Autodesk Fusion 360 part; units mm, degrees
(part 7 of 12)
  line L124 (13.462, -40.1221) -> (13.462, -36.3221)
  line L125 (17.262, -40.1221) -> (13.462, -40.1221)
  line L126 (13.462, -36.3221) -> (17.262, -36.3221)
  line L127 (17.262, -36.3221) -> (17.262, -40.1221)
  line L128 (52.9466, -41.1381) -> (49.1466, -41.1381)
  line L129 (49.1466, -41.1381) -> (49.1466, -37.3381)
  line L130 (49.1466, -37.3381) -> (52.9466, -37.3381)
  line L131 (52.9466, -37.3381) -> (52.9466, -41.1381)
  line L132 (-185.9511, -63.3791) -> (-185.9511, -67.1791)
  line L133 (-185.9511, -67.1791) -> (-189.7511, -67.1791)
  line L134 (-189.7511, -63.3791) -> (-185.9511, -63.3791)
  line L135 (-189.7511, -67.1791) -> (-189.7511, -63.3791)
  line L136 (-155.9511, -67.1791) -> (-159.7511, -67.1791)
  line L137 (-159.7511, -67.1791) -> (-159.7511, -63.3791)
  line L138 (-155.9511, -63.3791) -> (-155.9511, -67.1791)
  line L139 (-159.7511, -63.3791) -> (-155.9511, -63.3791)
  line L140 (-125.9511, -67.1791) -> (-129.7511, -67.1791)
  line L141 (-125.9511, -63.3791) -> (-125.9511, -67.1791)
  line L142 (-129.7511, -67.1791) -> (-129.7511, -63.3791)
  line L143 (-129.7511, -63.3791) -> (-125.9511, -63.3791)
  line L144 (-99.7511, -67.1791) -> (-99.7511, -63.3791)
  line L145 (-95.9511, -67.1791) -> (-99.7511, -67.1791)
  line L146 (-99.7511, -63.3791) -> (-95.9511, -63.3791)
  line L147 (-95.9511, -63.3791) -> (-95.9511, -67.1791)
  line L148 (-69.7511, -63.3791) -> (-65.9511, -63.3791)
  line L149 (-65.9511, -63.3791) -> (-65.9511, -67.1791)
  line L150 (-69.7511, -67.1791) -> (-69.7511, -63.3791)
  line L151 (-65.9511, -67.1791) -> (-69.7511, -67.1791)
  line L152 (-35.9511, -63.3791) -> (-35.9511, -67.1791)
  line L153 (-39.7511, -63.3791) -> (-35.9511, -63.3791)
  line L154 (-39.7511, -67.1791) -> (-39.7511, -63.3791)
  line L155 (-35.9511, -67.1791) -> (-39.7511, -67.1791)
  line L156 (6.975, -64.3891) -> (6.975, -68.1891)
  line L157 (3.175, -68.1891) -> (3.175, -64.3891)
  line L158 (3.175, -64.3891) -> (6.975, -64.3891)
  line L159 (6.975, -68.1891) -> (3.175, -68.1891)
  line L160 (-174.6989, -98.2882) -> (-178.4989, -98.2882)
  line L161 (-178.4989, -98.2882) -> (-178.4989, -94.4882)
  line L162 (-178.4989, -94.4882) -> (-174.6989, -94.4882)
  line L163 (-174.6989, -94.4882) -> (-174.6989, -98.2882)
  line L164 (52.0701, -75.5551) -> (52.0701, -71.7551)
  line L165 (55.8701, -71.7551) -> (55.8701, -75.5551)
  line L166 (55.8701, -75.5551) -> (52.0701, -75.5551)
  line L167 (52.0701, -71.7551) -> (55.8701, -71.7551)
  line L168 (-144.2823, -98.2882) -> (-148.0823, -98.2882)
  line L169 (-144.2823, -94.4882) -> (-144.2823, -98.2882)
  line L170 (-148.0823, -94.4882) -> (-144.2823, -94.4882)
  line L171 (-148.0823, -98.2882) -> (-148.0823, -94.4882)
  line L172 (-113.8658, -94.4882) -> (-113.8658, -98.2882)
  line L173 (-117.6658, -94.4882) -> (-113.8658, -94.4882)
  line L174 (-113.8658, -98.2882) -> (-117.6658, -98.2882)
  line L175 (-117.6658, -98.2882) -> (-117.6658, -94.4882)
  line L176 (-83.4492, -98.2882) -> (-87.2492, -98.2882)
  line L177 (-83.4492, -94.4882) -> (-83.4492, -98.2882)
  line L178 (-87.2492, -94.4882) -> (-83.4492, -94.4882)
  line L179 (-87.2492, -98.2882) -> (-87.2492, -94.4882)
  line L180 (-53.0326, -94.4882) -> (-53.0326, -98.2882)
  line L181 (-56.8326, -94.4882) -> (-53.0326, -94.4882)
  line L182 (-56.8326, -98.2882) -> (-56.8326, -94.4882)
  line L183 (-53.0326, -98.2882) -> (-56.8326, -98.2882)
  line L184 (-22.6161, -94.4882) -> (-22.6161, -98.2882)
  line L185 (-26.4161, -94.4882) -> (-22.6161, -94.4882)
  line L186 (-22.6161, -98.2882) -> (-26.4161, -98.2882)
  line L187 (-26.4161, -98.2882) -> (-26.4161, -94.4882)
  line L188 (7.737, -98.3894) -> (3.937, -98.3894)
  line L189 (3.937, -98.3894) -> (3.937, -94.5894)
  line L190 (7.737, -94.5894) -> (7.737, -98.3894)
  line L191 (3.937, -94.5894) -> (7.737, -94.5894)
  line L192 (-155.2293, -124.9242) -> (-155.2293, -128.7242)
  line L193 (-155.2293, -128.7242) -> (-159.0293, -128.7242)
  line L194 (-159.0293, -124.9242) -> (-155.2293, -124.9242)
  line L195 (-159.0293, -128.7242) -> (-159.0293, -124.9242)
  line L196 (-116.37, -124.9242) -> (-112.57, -124.9242)
  line L197 (-112.57, -124.9242) -> (-112.57, -128.7242)
  line L198 (-112.57, -128.7242) -> (-116.37, -128.7242)
  line L199 (-116.37, -128.7242) -> (-116.37, -124.9242)
  line L200 (-82.57, -128.7242) -> (-86.37, -128.7242)
  line L201 (-86.37, -128.7242) -> (-86.37, -124.9242)
  line L202 (-86.37, -124.9242) -> (-82.57, -124.9242)
  line L203 (-82.57, -124.9242) -> (-82.57, -128.7242)
  line L204 (-52.57, -128.7242) -> (-56.37, -128.7242)
  line L205 (-56.37, -128.7242) -> (-56.37, -124.9242)
  line L206 (-52.57, -124.9242) -> (-52.57, -128.7242)
  line L207 (-56.37, -124.9242) -> (-52.57, -124.9242)
  line L208 (-22.57, -124.9242) -> (-22.57, -128.7242)
  line L209 (-22.57, -128.7242) -> (-26.37, -128.7242)
  line L210 (-26.37, -124.9242) -> (-22.57, -124.9242)
  line L211 (-26.37, -128.7242) -> (-26.37, -124.9242)
  line L212 (3.63, -124.9242) -> (7.43, -124.9242)
  line L213 (7.43, -128.7242) -> (3.63, -128.7242)
  line L214 (7.43, -124.9242) -> (7.43, -128.7242)
  line L215 (3.63, -128.7242) -> (3.63, -124.9242)
  line L216 (33.63, -124.9242) -> (37.43, -124.9242)
  line L217 (37.43, -128.7242) -> (33.63, -128.7242)
  line L218 (33.63, -128.7242) -> (33.63, -124.9242)
  line L219 (37.43, -124.9242) -> (37.43, -128.7242)
  line L220 (66.8401, 26.2001) -> (66.8401, 24.6001)
  line L221 (65.2401, 24.6001) -> (65.2401, 26.2001)
  line L222 (65.2401, 26.2001) -> (66.8401, 26.2001)
  line L223 (66.8401, 24.6001) -> (65.2401, 24.6001)
  line L224 (66.8401, 24.6001) -> (65.2401, 24.6001)
  line L225 (65.2401, 24.6001) -> (65.2401, 26.2001)
  line L226 (65.2401, 26.2001) -> (66.8401, 26.2001)
  line L227 (66.8401, 26.2001) -> (66.8401, 24.6001)
  line L228 (65.2401, 24.6001) -> (65.2401, 26.2001)
  line L229 (66.8401, 26.2001) -> (66.8401, 24.6001)
  line L230 (65.2401, 26.2001) -> (66.8401, 26.2001)
  line L231 (66.8401, 24.6001) -> (65.2401, 24.6001)
  arc A292 (65.2401, 22.86) -> (66.8401, 22.86) centre (66.0401, 22.86) ccw
  arc A293 (66.8401, 22.86) -> (65.2401, 22.86) centre (66.0401, 22.86) ccw
  arc A294 (65.2401, 22.86) -> (66.8401, 22.86) centre (66.0401, 22.86) ccw
  arc A295 (66.8401, 22.86) -> (65.2401, 22.86) centre (66.0401, 22.86) ccw
  arc A296 (66.8401, 22.86) -> (65.2401, 22.86) centre (66.0401, 22.86) ccw
  arc A297 (65.2401, 22.86) -> (66.8401, 22.86) centre (66.0401, 22.86) ccw
  arc A298 (66.8401, 20.32) -> (65.2401, 20.32) centre (66.0401, 20.32) ccw
  arc A299 (65.2401, 20.32) -> (66.8401, 20.32) centre (66.0401, 20.32) ccw
  arc A300 (65.2401, 20.32) -> (66.8401, 20.32) centre (66.0401, 20.32) ccw
  arc A301 (66.8401, 20.32) -> (65.2401, 20.32) centre (66.0401, 20.32) ccw
  arc A302 (65.2401, 20.32) -> (66.8401, 20.32) centre (66.0401, 20.32) ccw
  arc A303 (66.8401, 20.32) -> (65.2401, 20.32) centre (66.0401, 20.32) ccw
  arc A304 (65.2401, 17.78) -> (66.8401, 17.78) centre (66.0401, 17.78) ccw
  arc A305 (66.8401, 17.78) -> (65.2401, 17.78) centre (66.0401, 17.78) ccw
  arc A306 (65.2401, 17.78) -> (66.8401, 17.78) centre (66.0401, 17.78) ccw
  arc A307 (66.8401, 17.78) -> (65.2401, 17.78) centre (66.0401, 17.78) ccw
  arc A308 (66.8401, 17.78) -> (65.2401, 17.78) centre (66.0401, 17.78) ccw
  arc A309 (65.2401, 17.78) -> (66.8401, 17.78) centre (66.0401, 17.78) ccw
  arc A310 (66.8401, 15.24) -> (65.2401, 15.24) centre (66.0401, 15.24) ccw
  arc A311 (65.2401, 15.24) -> (66.8401, 15.24) centre (66.0401, 15.24) ccw
  arc A312 (65.2401, 15.24) -> (66.8401, 15.24) centre (66.0401, 15.24) ccw
  arc A313 (66.8401, 15.24) -> (65.2401, 15.24) centre (66.0401, 15.24) ccw
  arc A314 (66.8401, 15.24) -> (65.2401, 15.24) centre (66.0401, 15.24) ccw
  arc A315 (65.2401, 15.24) -> (66.8401, 15.24) centre (66.0401, 15.24) ccw
  arc A316 (66.8401, 12.7) -> (65.2401, 12.7) centre (66.0401, 12.7) ccw
  arc A317 (65.2401, 12.7) -> (66.8401, 12.7) centre (66.0401, 12.7) ccw
  arc A318 (65.2401, 12.7) -> (66.8401, 12.7) centre (66.0401, 12.7) ccw
  arc A319 (66.8401, 12.7) -> (65.2401, 12.7) centre (66.0401, 12.7) ccw
  arc A320 (66.8401, 12.7) -> (65.2401, 12.7) centre (66.0401, 12.7) ccw
  arc A321 (65.2401, 12.7) -> (66.8401, 12.7) centre (66.0401, 12.7) ccw
  arc A322 (66.8401, 10.16) -> (65.2401, 10.16) centre (66.0401, 10.16) ccw
  arc A323 (65.2401, 10.16) -> (66.8401, 10.16) centre (66.0401, 10.16) ccw
  arc A324 (65.2401, 10.16) -> (66.8401, 10.16) centre (66.0401, 10.16) ccw
  arc A325 (66.8401, 10.16) -> (65.2401, 10.16) centre (66.0401, 10.16) ccw
  arc A326 (66.8401, 10.16) -> (65.2401, 10.16) centre (66.0401, 10.16) ccw
  arc A327 (65.2401, 10.16) -> (66.8401, 10.16) centre (66.0401, 10.16) ccw
  arc A328 (66.8401, 7.62) -> (65.2401, 7.62) centre (66.0401, 7.62) ccw
  arc A329 (65.2401, 7.62) -> (66.8401, 7.62) centre (66.0401, 7.62) ccw
  arc A330 (66.8401, 7.62) -> (65.2401, 7.62) centre (66.0401, 7.62) ccw
  arc A331 (65.2401, 7.62) -> (66.8401, 7.62) centre (66.0401, 7.62) ccw
  arc A332 (66.8401, 7.62) -> (65.2401, 7.62) centre (66.0401, 7.62) ccw
  arc A333 (65.2401, 7.62) -> (66.8401, 7.62) centre (66.0401, 7.62) ccw
  arc A334 (65.2401, 5.08) -> (66.8401, 5.08) centre (66.0401, 5.08) ccw
  arc A335 (66.8401, 5.08) -> (65.2401, 5.08) centre (66.0401, 5.08) ccw
  arc A336 (66.8401, 5.08) -> (65.2401, 5.08) centre (66.0401, 5.08) ccw
  arc A337 (65.2401, 5.08) -> (66.8401, 5.08) centre (66.0401, 5.08) ccw
  arc A338 (65.2401, 5.08) -> (66.8401, 5.08) centre (66.0401, 5.08) ccw
  arc A339 (66.8401, 5.08) -> (65.2401, 5.08) centre (66.0401, 5.08) ccw
  arc A340 (65.2401, 2.54) -> (66.8401, 2.54) centre (66.0401, 2.54) ccw
  arc A341 (66.8401, 2.54) -> (65.2401, 2.54) centre (66.0401, 2.54) ccw
  arc A342 (65.2401, 2.54) -> (66.8401, 2.54) centre (66.0401, 2.54) ccw
  arc A343 (66.8401, 2.54) -> (65.2401, 2.54) centre (66.0401, 2.54) ccw
  arc A344 (66.8401, 2.54) -> (65.2401, 2.54) centre (66.0401, 2.54) ccw
  arc A345 (65.2401, 2.54) -> (66.8401, 2.54) centre (66.0401, 2.54) ccw
  arc A346 (66.8401, 0) -> (65.2401, 0) centre (66.0401, 0) ccw
  arc A347 (65.2401, 0) -> (66.8401, 0) centre (66.0401, 0) ccw
  arc A348 (65.2401, 0) -> (66.8401, 0) centre (66.0401, 0) ccw
  arc A349 (66.8401, 0) -> (65.2401, 0) centre (66.0401, 0) ccw
  arc A350 (65.2401, 0) -> (66.8401, 0) centre (66.0401, 0) ccw
  arc A351 (66.8401, 0) -> (65.2401, 0) centre (66.0401, 0) ccw
  arc A352 (65.2401, -2.54) -> (66.8401, -2.54) centre (66.0401, -2.54) ccw
  arc A353 (66.8401, -2.54) -> (65.2401, -2.54) centre (66.0401, -2.54) ccw
  arc A354 (65.2401, -2.54) -> (66.8401, -2.54) centre (66.0401, -2.54) ccw
  arc A355 (66.8401, -2.54) -> (65.2401, -2.54) centre (66.0401, -2.54) ccw
  arc A356 (66.8401, -2.54) -> (65.2401, -2.54) centre (66.0401, -2.54) ccw
  arc A357 (65.2401, -2.54) -> (66.8401, -2.54) centre (66.0401, -2.54) ccw
  arc A358 (66.8401, -5.08) -> (65.2401, -5.08) centre (66.0401, -5.08) ccw
  arc A359 (65.2401, -5.08) -> (66.8401, -5.08) centre (66.0401, -5.08) ccw
  arc A360 (66.8401, -5.08) -> (65.2401, -5.08) centre (66.0401, -5.08) ccw
  arc A361 (65.2401, -5.08) -> (66.8401, -5.08) centre (66.0401, -5.08) ccw
  arc A362 (66.8401, -5.08) -> (65.2401, -5.08) centre (66.0401, -5.08) ccw
  arc A363 (65.2401, -5.08) -> (66.8401, -5.08) centre (66.0401, -5.08) ccw
  arc A364 (65.2401, -7.62) -> (66.8401, -7.62) centre (66.0401, -7.62) ccw
  arc A365 (66.8401, -7.62) -> (65.2401, -7.62) centre (66.0401, -7.62) ccw
  arc A366 (66.8401, -7.62) -> (65.2401, -7.62) centre (66.0401, -7.62) ccw
  arc A367 (65.2401, -7.62) -> (66.8401, -7.62) centre (66.0401, -7.62) ccw
  arc A368 (66.8401, -7.62) -> (65.2401, -7.62) centre (66.0401, -7.62) ccw
  arc A369 (65.2401, -7.62) -> (66.8401, -7.62) centre (66.0401, -7.62) ccw
  arc A370 (65.2401, -10.16) -> (66.8401, -10.16) centre (66.0401, -10.16) ccw
  arc A371 (66.8401, -10.16) -> (65.2401, -10.16) centre (66.0401, -10.16) ccw
  arc A372 (65.2401, -10.16) -> (66.8401, -10.16) centre (66.0401, -10.16) ccw
  arc A373 (66.8401, -10.16) -> (65.2401, -10.16) centre (66.0401, -10.16) ccw
  arc A374 (65.2401, -10.16) -> (66.8401, -10.16) centre (66.0401, -10.16) ccw
  arc A375 (66.8401, -10.16) -> (65.2401, -10.16) centre (66.0401, -10.16) ccw
  arc A376 (65.2401, -12.7) -> (66.8401, -12.7) centre (66.0401, -12.7) ccw
  arc A377 (66.8401, -12.7) -> (65.2401, -12.7) centre (66.0401, -12.7) ccw
  arc A378 (65.2401, -12.7) -> (66.8401, -12.7) centre (66.0401, -12.7) ccw
  arc A379 (66.8401, -12.7) -> (65.2401, -12.7) centre (66.0401, -12.7) ccw
  arc A380 (66.8401, -12.7) -> (65.2401, -12.7) centre (66.0401, -12.7) ccw
  arc A381 (65.2401, -12.7) -> (66.8401, -12.7) centre (66.0401, -12.7) ccw
  arc A382 (66.8328, -15.2362) -> (65.2328, -15.2362) centre (66.0328, -15.2362) ccw
  arc A383 (65.2328, -15.2362) -> (66.8328, -15.2362) centre (66.0328, -15.2362) ccw
  arc A384 (65.2328, -15.2362) -> (66.8328, -15.2362) centre (66.0328, -15.2362) ccw
  arc A385 (66.8328, -15.2362) -> (65.2328, -15.2362) centre (66.0328, -15.2362) ccw
  arc A386 (66.8328, -15.2362) -> (65.2328, -15.2362) centre (66.0328, -15.2362) ccw
  arc A387 (65.2328, -15.2362) -> (66.8328, -15.2362) centre (66.0328, -15.2362) ccw
  arc A388 (66.8401, -17.78) -> (65.2401, -17.78) centre (66.0401, -17.78) ccw
  arc A389 (65.2401, -17.78) -> (66.8401, -17.78) centre (66.0401, -17.78) ccw
  arc A390 (66.8401, -17.78) -> (65.2401, -17.78) centre (66.0401, -17.78) ccw
  arc A391 (65.2401, -17.78) -> (66.8401, -17.78) centre (66.0401, -17.78) ccw
  arc A392 (66.8401, -17.78) -> (65.2401, -17.78) centre (66.0401, -17.78) ccw
  arc A393 (65.2401, -17.78) -> (66.8401, -17.78) centre (66.0401, -17.78) ccw
  arc A394 (65.2401, -20.32) -> (66.8401, -20.32) centre (66.0401, -20.32) ccw
  arc A395 (66.8401, -20.32) -> (65.2401, -20.32) centre (66.0401, -20.32) ccw
  arc A396 (65.2401, -20.32) -> (66.8401, -20.32) centre (66.0401, -20.32) ccw
  arc A397 (66.8401, -20.32) -> (65.2401, -20.32) centre (66.0401, -20.32) ccw
  arc A398 (66.8401, -20.32) -> (65.2401, -20.32) centre (66.0401, -20.32) ccw
  arc A399 (65.2401, -20.32) -> (66.8401, -20.32) centre (66.0401, -20.32) ccw
  arc A400 (65.2401, -22.86) -> (66.8401, -22.86) centre (66.0401, -22.86) ccw
  arc A401 (66.8401, -22.86) -> (65.2401, -22.86) centre (66.0401, -22.86) ccw
  arc A402 (66.8401, -22.86) -> (65.2401, -22.86) centre (66.0401, -22.86) ccw
  arc A403 (65.2401, -22.86) -> (66.8401, -22.86) centre (66.0401, -22.86) ccw
  arc A404 (65.2401, -22.86) -> (66.8401, -22.86) centre (66.0401, -22.86) ccw
  arc A405 (66.8401, -22.86) -> (65.2401, -22.86) centre (66.0401, -22.86) ccw
  arc A406 (84.6202, -22.86) -> (83.0202, -22.86) centre (83.8202, -22.86) ccw
  arc A407 (83.0202, -22.86) -> (84.6202, -22.86) centre (83.8202, -22.86) ccw
  arc A408 (84.6202, -22.86) -> (83.0202, -22.86) centre (83.8202, -22.86) ccw
  arc A409 (83.0202, -22.86) -> (84.6202, -22.86) centre (83.8202, -22.86) ccw
  arc A410 (83.0202, -22.86) -> (84.6202, -22.86) centre (83.8202, -22.86) ccw
  arc A411 (84.6202, -22.86) -> (83.0202, -22.86) centre (83.8202, -22.86) ccw
  arc A412 (84.6202, -20.32) -> (83.0202, -20.32) centre (83.8202, -20.32) ccw
  arc A413 (83.0202, -20.32) -> (84.6202, -20.32) centre (83.8202, -20.32) ccw
  arc A414 (84.6202, -20.32) -> (83.0202, -20.32) centre (83.8202, -20.32) ccw
  arc A415 (83.0202, -20.32) -> (84.6202, -20.32) centre (83.8202, -20.32) ccw
  arc A416 (84.6202, -20.32) -> (83.0202, -20.32) centre (83.8202, -20.32) ccw
  arc A417 (83.0202, -20.32) -> (84.6202, -20.32) centre (83.8202, -20.32) ccw
  arc A418 (83.0202, -17.8517) -> (84.6202, -17.8517) centre (83.8202, -17.8517) ccw
  arc A419 (84.6202, -17.8517) -> (83.0202, -17.8517) centre (83.8202, -17.8517) ccw
  arc A420 (83.0202, -17.8517) -> (84.6202, -17.8517) centre (83.8202, -17.8517) ccw
  arc A421 (84.6202, -17.8517) -> (83.0202, -17.8517) centre (83.8202, -17.8517) ccw
  arc A422 (83.0202, -17.8517) -> (84.6202, -17.8517) centre (83.8202, -17.8517) ccw
  arc A423 (84.6202, -17.8517) -> (83.0202, -17.8517) centre (83.8202, -17.8517) ccw
  arc A424 (83.0202, -15.24) -> (84.6202, -15.24) centre (83.8202, -15.24) ccw
  arc A425 (84.6202, -15.24) -> (83.0202, -15.24) centre (83.8202, -15.24) ccw
  arc A426 (84.6202, -15.24) -> (83.0202, -15.24) centre (83.8202, -15.24) ccw
  arc A427 (83.0202, -15.24) -> (84.6202, -15.24) centre (83.8202, -15.24) ccw
  arc A428 (84.6202, -15.24) -> (83.0202, -15.24) centre (83.8202, -15.24) ccw
  arc A429 (83.0202, -15.24) -> (84.6202, -15.24) centre (83.8202, -15.24) ccw
  arc A430 (84.6202, -12.7) -> (83.0202, -12.7) centre (83.8202, -12.7) ccw
  arc A431 (83.0202, -12.7) -> (84.6202, -12.7) centre (83.8202, -12.7) ccw
  arc A432 (84.6202, -12.7) -> (83.0202, -12.7) centre (83.8202, -12.7) ccw
  arc A433 (83.0202, -12.7) -> (84.6202, -12.7) centre (83.8202, -12.7) ccw
  arc A434 (83.0202, -12.7) -> (84.6202, -12.7) centre (83.8202, -12.7) ccw
  arc A435 (84.6202, -12.7) -> (83.0202, -12.7) centre (83.8202, -12.7) ccw
  arc A436 (84.6202, -10.16) -> (83.0202, -10.16) centre (83.8202, -10.16) ccw
  arc A437 (83.0202, -10.16) -> (84.6202, -10.16) centre (83.8202, -10.16) ccw
  arc A438 (83.0202, -10.16) -> (84.6202, -10.16) centre (83.8202, -10.16) ccw
  arc A439 (84.6202, -10.16) -> (83.0202, -10.16) centre (83.8202, -10.16) ccw
  arc A440 (83.0202, -10.16) -> (84.6202, -10.16) centre (83.8202, -10.16) ccw
  arc A441 (84.6202, -10.16) -> (83.0202, -10.16) centre (83.8202, -10.16) ccw
  arc A442 (83.0202, -7.62) -> (84.6202, -7.62) centre (83.8202, -7.62) ccw
  arc A443 (84.6202, -7.62) -> (83.0202, -7.62) centre (83.8202, -7.62) ccw
  arc A444 (83.0202, -7.62) -> (84.6202, -7.62) centre (83.8202, -7.62) ccw
  arc A445 (84.6202, -7.62) -> (83.0202, -7.62) centre (83.8202, -7.62) ccw
  arc A446 (83.0202, -7.62) -> (84.6202, -7.62) centre (83.8202, -7.62) ccw
  arc A447 (84.6202, -7.62) -> (83.0202, -7.62) centre (83.8202, -7.62) ccw
  arc A448 (84.6202, -5.08) -> (83.0202, -5.08) centre (83.8202, -5.08) ccw
  arc A449 (83.0202, -5.08) -> (84.6202, -5.08) centre (83.8202, -5.08) ccw
  arc A450 (83.0202, -5.08) -> (84.6202, -5.08) centre (83.8202, -5.08) ccw
  arc A451 (84.6202, -5.08) -> (83.0202, -5.08) centre (83.8202, -5.08) ccw
  arc A452 (83.0202, -5.08) -> (84.6202, -5.08) centre (83.8202, -5.08) ccw
  arc A453 (84.6202, -5.08) -> (83.0202, -5.08) centre (83.8202, -5.08) ccw
  arc A454 (83.0202, -2.54) -> (84.6202, -2.54) centre (83.8202, -2.54) ccw
  arc A455 (84.6202, -2.54) -> (83.0202, -2.54) centre (83.8202, -2.54) ccw
  arc A456 (83.0202, -2.54) -> (84.6202, -2.54) centre (83.8202, -2.54) ccw
  arc A457 (84.6202, -2.54) -> (83.0202, -2.54) centre (83.8202, -2.54) ccw
  arc A458 (84.6202, -2.54) -> (83.0202, -2.54) centre (83.8202, -2.54) ccw
  arc A459 (83.0202, -2.54) -> (84.6202, -2.54) centre (83.8202, -2.54) ccw
  arc A460 (84.6202, 0) -> (83.0202, 0) centre (83.8202, 0) ccw
  arc A461 (83.0202, 0) -> (84.6202, 0) centre (83.8202, 0) ccw
  arc A462 (84.6202, 0) -> (83.0202, 0) centre (83.8202, 0) ccw
  arc A463 (83.0202, 0) -> (84.6202, 0) centre (83.8202, 0) ccw
  arc A464 (83.0202, 0) -> (84.6202, 0) centre (83.8202, 0) ccw
  arc A465 (84.6202, 0) -> (83.0202, 0) centre (83.8202, 0) ccw
  arc A466 (83.0202, 2.54) -> (84.6202, 2.54) centre (83.8202, 2.54) ccw
  arc A467 (84.6202, 2.54) -> (83.0202, 2.54) centre (83.8202, 2.54) ccw
  arc A468 (83.0202, 2.54) -> (84.6202, 2.54) centre (83.8202, 2.54) ccw
  arc A469 (84.6202, 2.54) -> (83.0202, 2.54) centre (83.8202, 2.54) ccw
  arc A470 (83.0202, 2.54) -> (84.6202, 2.54) centre (83.8202, 2.54) ccw
  arc A471 (84.6202, 2.54) -> (83.0202, 2.54) centre (83.8202, 2.54) ccw
  arc A472 (84.6202, 5.08) -> (83.0202, 5.08) centre (83.8202, 5.08) ccw
  arc A473 (83.0202, 5.08) -> (84.6202, 5.08) centre (83.8202, 5.08) ccw
  arc A474 (84.6202, 5.08) -> (83.0202, 5.08) centre (83.8202, 5.08) ccw
  arc A475 (83.0202, 5.08) -> (84.6202, 5.08) centre (83.8202, 5.08) ccw
  arc A476 (83.0202, 5.08) -> (84.6202, 5.08) centre (83.8202, 5.08) ccw
  arc A477 (84.6202, 5.08) -> (83.0202, 5.08) centre (83.8202, 5.08) ccw
  arc A478 (83.0202, 7.62) -> (84.6202, 7.62) centre (83.8202, 7.62) ccw
  arc A479 (84.6202, 7.62) -> (83.0202, 7.62) centre (83.8202, 7.62) ccw
  arc A480 (83.0202, 7.62) -> (84.6202, 7.62) centre (83.8202, 7.62) ccw
  arc A481 (84.6202, 7.62) -> (83.0202, 7.62) centre (83.8202, 7.62) ccw
  arc A482 (84.6202, 7.62) -> (83.0202, 7.62) centre (83.8202, 7.62) ccw
  arc A483 (83.0202, 7.62) -> (84.6202, 7.62) centre (83.8202, 7.62) ccw
  arc A484 (83.0202, 10.16) -> (84.6202, 10.16) centre (83.8202, 10.16) ccw
  arc A485 (84.6202, 10.16) -> (83.0202, 10.16) centre (83.8202, 10.16) ccw
  arc A486 (83.0202, 10.16) -> (84.6202, 10.16) centre (83.8202, 10.16) ccw
  arc A487 (84.6202, 10.16) -> (83.0202, 10.16) centre (83.8202, 10.16) ccw
  arc A488 (83.0202, 10.16) -> (84.6202, 10.16) centre (83.8202, 10.16) ccw
  arc A489 (84.6202, 10.16) -> (83.0202, 10.16) centre (83.8202, 10.16) ccw
  arc A490 (84.6202, 12.7) -> (83.0202, 12.7) centre (83.8202, 12.7) ccw
  arc A491 (83.0202, 12.7) -> (84.6202, 12.7) centre (83.8202, 12.7) ccw
  arc A492 (83.0202, 12.7) -> (84.6202, 12.7) centre (83.8202, 12.7) ccw
  arc A493 (84.6202, 12.7) -> (83.0202, 12.7) centre (83.8202, 12.7) ccw
  arc A494 (83.0202, 12.7) -> (84.6202, 12.7) centre (83.8202, 12.7) ccw
  arc A495 (84.6202, 12.7) -> (83.0202, 12.7) centre (83.8202, 12.7) ccw
  arc A496 (84.6202, 15.24) -> (83.0202, 15.24) centre (83.8202, 15.24) ccw
  arc A497 (83.0202, 15.24) -> (84.6202, 15.24) centre (83.8202, 15.24) ccw
  arc A498 (84.6202, 15.24) -> (83.0202, 15.24) centre (83.8202, 15.24) ccw
  arc A499 (83.0202, 15.24) -> (84.6202, 15.24) centre (83.8202, 15.24) ccw
  arc A500 (83.0202, 15.24) -> (84.6202, 15.24) centre (83.8202, 15.24) ccw
  arc A501 (84.6202, 15.24) -> (83.0202, 15.24) centre (83.8202, 15.24) ccw
  arc A502 (84.6202, 17.78) -> (83.0202, 17.78) centre (83.8202, 17.78) ccw
  arc A503 (83.0202, 17.78) -> (84.6202, 17.78) centre (83.8202, 17.78) ccw
  arc A504 (84.6202, 17.78) -> (83.0202, 17.78) centre (83.8202, 17.78) ccw
  arc A505 (83.0202, 17.78) -> (84.6202, 17.78) centre (83.8202, 17.78) ccw
  arc A506 (83.0202, 17.78) -> (84.6202, 17.78) centre (83.8202, 17.78) ccw
  arc A507 (84.6202, 17.78) -> (83.0202, 17.78) centre (83.8202, 17.78) ccw
  arc A508 (84.6202, 20.32) -> (83.0202, 20.32) centre (83.8202, 20.32) ccw
  arc A509 (83.0202, 20.32) -> (84.6202, 20.32) centre (83.8202, 20.32) ccw
  arc A510 (83.0202, 20.32) -> (84.6202, 20.32) centre (83.8202, 20.32) ccw
  arc A511 (84.6202, 20.32) -> (83.0202, 20.32) centre (83.8202, 20.32) ccw
  arc A512 (84.6202, 20.32) -> (83.0202, 20.32) centre (83.8202, 20.32) ccw
  arc A513 (83.0202, 20.32) -> (84.6202, 20.32) centre (83.8202, 20.32) ccw
  arc A514 (84.6202, 22.86) -> (83.0202, 22.86) centre (83.8202, 22.86) ccw
  arc A515 (83.0202, 22.86) -> (84.6202, 22.86) centre (83.8202, 22.86) ccw
  arc A516 (83.0202, 22.86) -> (84.6202, 22.86) centre (83.8202, 22.86) ccw
  arc A517 (84.6202, 22.86) -> (83.0202, 22.86) centre (83.8202, 22.86) ccw
  arc A518 (84.6202, 22.86) -> (83.0202, 22.86) centre (83.8202, 22.86) ccw
  arc A519 (83.0202, 22.86) -> (84.6202, 22.86) centre (83.8202, 22.86) ccw
  arc A520 (84.6202, 25.4001) -> (83.0202, 25.4001) centre (83.8202, 25.4001) ccw
  arc A521 (83.0202, 25.4001) -> (84.6202, 25.4001) centre (83.8202, 25.4001) ccw
  arc A522 (83.0202, 25.4001) -> (84.6202, 25.4001) centre (83.8202, 25.4001) ccw
  arc A523 (84.6202, 25.4001) -> (83.0202, 25.4001) centre (83.8202, 25.4001) ccw
  arc A524 (83.0202, 25.4001) -> (84.6202, 25.4001) centre (83.8202, 25.4001) ccw
  arc A525 (84.6202, 25.4001) -> (83.0202, 25.4001) centre (83.8202, 25.4001) ccw
  arc A526 (71.9201, -22.86) -> (70.3201, -22.86) centre (71.1201, -22.86) ccw
  arc A527 (70.3201, -22.86) -> (71.9201, -22.86) centre (71.1201, -22.86) ccw
  arc A528 (70.3201, -22.86) -> (71.9201, -22.86) centre (71.1201, -22.86) ccw
  arc A529 (71.9201, -22.86) -> (70.3201, -22.86) centre (71.1201, -22.86) ccw
  arc A530 (71.9201, -22.86) -> (70.3201, -22.86) centre (71.1201, -22.86) ccw
  arc A531 (70.3201, -22.86) -> (71.9201, -22.86) centre (71.1201, -22.86) ccw
  arc A532 (74.4601, -22.86) -> (72.8601, -22.86) centre (73.6601, -22.86) ccw
  arc A533 (72.8601, -22.86) -> (74.4601, -22.86) centre (73.6601, -22.86) ccw
  arc A534 (72.8601, -22.86) -> (74.4601, -22.86) centre (73.6601, -22.86) ccw
  arc A535 (74.4601, -22.86) -> (72.8601, -22.86) centre (73.6601, -22.86) ccw
  arc A536 (72.8601, -22.86) -> (74.4601, -22.86) centre (73.6601, -22.86) ccw
  arc A537 (74.4601, -22.86) -> (72.8601, -22.86) centre (73.6601, -22.86) ccw
  arc A538 (77.0002, -22.86) -> (75.4002, -22.86) centre (76.2002, -22.86) ccw
  arc A539 (75.4002, -22.86) -> (77.0002, -22.86) centre (76.2002, -22.86) ccw
  arc A540 (75.4002, -22.86) -> (77.0002, -22.86) centre (76.2002, -22.86) ccw
  arc A541 (77.0002, -22.86) -> (75.4002, -22.86) centre (76.2002, -22.86) ccw
  arc A542 (77.0002, -22.86) -> (75.4002, -22.86) centre (76.2002, -22.86) ccw
  arc A543 (75.4002, -22.86) -> (77.0002, -22.86) centre (76.2002, -22.86) ccw
  arc A544 (79.5402, -22.86) -> (77.9402, -22.86) centre (78.7402, -22.86) ccw
  arc A545 (77.9402, -22.86) -> (79.5402, -22.86) centre (78.7402, -22.86) ccw
  arc A546 (79.5402, -22.86) -> (77.9402, -22.86) centre (78.7402, -22.86) ccw
  arc A547 (77.9402, -22.86) -> (79.5402, -22.86) centre (78.7402, -22.86) ccw
  arc A548 (79.5402, -22.86) -> (77.9402, -22.86) centre (78.7402, -22.86) ccw
  arc A549 (77.9402, -22.86) -> (79.5402, -22.86) centre (78.7402, -22.86) ccw
  arc A550 (-178.73, 30) -> (-181.27, 30) centre (-180, 30) ccw
  arc A551 (-181.27, 30) -> (-178.73, 30) centre (-180, 30) ccw
  arc A552 (-181.27, 30) -> (-178.73, 30) centre (-180, 30) ccw
  arc A553 (-178.73, 30) -> (-181.27, 30) centre (-180, 30) ccw
  arc A554 (-181.27, 30) -> (-178.73, 30) centre (-180, 30) ccw
  arc A555 (-178.73, 30) -> (-181.27, 30) centre (-180, 30) ccw
  arc A556 (-185.08, 27.46) -> (-187.62, 27.46) centre (-186.35, 27.46) ccw
  arc A557 (-187.62, 27.46) -> (-185.08, 27.46) centre (-186.35, 27.46) ccw
  arc A558 (-185.08, 27.46) -> (-187.62, 27.46) centre (-186.35, 27.46) ccw
  arc A559 (-187.62, 27.46) -> (-185.08, 27.46) centre (-186.35, 27.46) ccw
  arc A560 (-187.62, 27.46) -> (-185.08, 27.46) centre (-186.35, 27.46) ccw
  arc A561 (-185.08, 27.46) -> (-187.62, 27.46) centre (-186.35, 27.46) ccw
  arc A562 (-148.73, 30) -> (-151.27, 30) centre (-150, 30) ccw
  arc A563 (-151.27, 30) -> (-148.73, 30) centre (-150, 30) ccw
  arc A564 (-151.27, 30) -> (-148.73, 30) centre (-150, 30) ccw
  arc A565 (-148.73, 30) -> (-151.27, 30) centre (-150, 30) ccw
  arc A566 (-148.73, 30) -> (-151.27, 30) centre (-150, 30) ccw
  arc A567 (-151.27, 30) -> (-148.73, 30) centre (-150, 30) ccw
  arc A568 (-155.08, 27.46) -> (-157.62, 27.46) centre (-156.35, 27.46) ccw
  arc A569 (-157.62, 27.46) -> (-155.08, 27.46) centre (-156.35, 27.46) ccw
  arc A570 (-157.62, 27.46) -> (-155.08, 27.46) centre (-156.35, 27.46) ccw
  arc A571 (-155.08, 27.46) -> (-157.62, 27.46) centre (-156.35, 27.46) ccw
  arc A572 (-157.62, 27.46) -> (-155.08, 27.46) centre (-156.35, 27.46) ccw
  arc A573 (-155.08, 27.46) -> (-157.62, 27.46) centre (-156.35, 27.46) ccw
  arc A574 (-121.27, 30) -> (-118.73, 30) centre (-120, 30) ccw
  arc A575 (-118.73, 30) -> (-121.27, 30) centre (-120, 30) ccw
  arc A576 (-121.27, 30) -> (-118.73, 30) centre (-120, 30) ccw
  arc A577 (-118.73, 30) -> (-121.27, 30) centre (-120, 30) ccw
  arc A578 (-121.27, 30) -> (-118.73, 30) centre (-120, 30) ccw
  arc A579 (-118.73, 30) -> (-121.27, 30) centre (-120, 30) ccw
  arc A580 (-125.08, 27.46) -> (-127.62, 27.46) centre (-126.35, 27.46) ccw
  arc A581 (-127.62, 27.46) -> (-125.08, 27.46) centre (-126.35, 27.46) ccw
  arc A582 (-127.62, 27.46) -> (-125.08, 27.46) centre (-126.35, 27.46) ccw
  arc A583 (-125.08, 27.46) -> (-127.62, 27.46) centre (-126.35, 27.46) ccw
  arc A584 (-125.08, 27.46) -> (-127.62, 27.46) centre (-126.35, 27.46) ccw
  arc A585 (-127.62, 27.46) -> (-125.08, 27.46) centre (-126.35, 27.46) ccw
  arc A586 (-88.73, 30) -> (-91.27, 30) centre (-90, 30) ccw
  arc A587 (-91.27, 30) -> (-88.73, 30) centre (-90, 30) ccw
  arc A588 (-88.73, 30) -> (-91.27, 30) centre (-90, 30) ccw
  arc A589 (-91.27, 30) -> (-88.73, 30) centre (-90, 30) ccw
  arc A590 (-88.73, 30) -> (-91.27, 30) centre (-90, 30) ccw
  arc A591 (-91.27, 30) -> (-88.73, 30) centre (-90, 30) ccw
  arc A592 (-95.08, 27.46) -> (-97.62, 27.46) centre (-96.35, 27.46) ccw
  arc A593 (-97.62, 27.46) -> (-95.08, 27.46) centre (-96.35, 27.46) ccw
  arc A594 (-95.08, 27.46) -> (-97.62, 27.46) centre (-96.35, 27.46) ccw
  arc A595 (-97.62, 27.46) -> (-95.08, 27.46) centre (-96.35, 27.46) ccw
  arc A596 (-95.08, 27.46) -> (-97.62, 27.46) centre (-96.35, 27.46) ccw
  arc A597 (-97.62, 27.46) -> (-95.08, 27.46) centre (-96.35, 27.46) ccw
  arc A598 (-61.27, 30) -> (-58.73, 30) centre (-60, 30) ccw
  arc A599 (-58.73, 30) -> (-61.27, 30) centre (-60, 30) ccw
  arc A600 (-61.27, 30) -> (-58.73, 30) centre (-60, 30) ccw
  arc A601 (-58.73, 30) -> (-61.27, 30) centre (-60, 30) ccw
  arc A602 (-58.73, 30) -> (-61.27, 30) centre (-60, 30) ccw
  arc A603 (-61.27, 30) -> (-58.73, 30) centre (-60, 30) ccw
  arc A604 (-65.08, 27.46) -> (-67.62, 27.46) centre (-66.35, 27.46) ccw
  arc A605 (-67.62, 27.46) -> (-65.08, 27.46) centre (-66.35, 27.46) ccw
  arc A606 (-67.62, 27.46) -> (-65.08, 27.46) centre (-66.35, 27.46) ccw
  arc A607 (-65.08, 27.46) -> (-67.62, 27.46) centre (-66.35, 27.46) ccw
  arc A608 (-67.62, 27.46) -> (-65.08, 27.46) centre (-66.35, 27.46) ccw
  arc A609 (-65.08, 27.46) -> (-67.62, 27.46) centre (-66.35, 27.46) ccw
  arc A610 (-31.27, 30) -> (-28.73, 30) centre (-30, 30) ccw
  arc A611 (-28.73, 30) -> (-31.27, 30) centre (-30, 30) ccw
  arc A612 (-28.73, 30) -> (-31.27, 30) centre (-30, 30) ccw
  arc A613 (-31.27, 30) -> (-28.73, 30) centre (-30, 30) ccw
  arc A614 (-28.73, 30) -> (-31.27, 30) centre (-30, 30) ccw
  arc A615 (-31.27, 30) -> (-28.73, 30) centre (-30, 30) ccw
  arc A616 (-37.62, 27.46) -> (-35.08, 27.46) centre (-36.35, 27.46) ccw
  arc A617 (-35.08, 27.46) -> (-37.62, 27.46) centre (-36.35, 27.46) ccw
  arc A618 (-35.08, 27.46) -> (-37.62, 27.46) centre (-36.35, 27.46) ccw
  arc A619 (-37.62, 27.46) -> (-35.08, 27.46) centre (-36.35, 27.46) ccw
  arc A620 (-35.08, 27.46) -> (-37.62, 27.46) centre (-36.35, 27.46) ccw
  arc A621 (-37.62, 27.46) -> (-35.08, 27.46) centre (-36.35, 27.46) ccw
  arc A622 (1.27, 30) -> (-1.27, 30) centre (0, 30) ccw
  arc A623 (-1.27, 30) -> (1.27, 30) centre (0, 30) ccw
  arc A624 (1.27, 30) -> (-1.27, 30) centre (0, 30) ccw
  arc A625 (-1.27, 30) -> (1.27, 30) centre (0, 30) ccw
  arc A626 (1.27, 30) -> (-1.27, 30) centre (0, 30) ccw
  arc A627 (-1.27, 30) -> (1.27, 30) centre (0, 30) ccw
  arc A628 (-5.08, 27.46) -> (-7.62, 27.46) centre (-6.35, 27.46) ccw
  arc A629 (-7.62, 27.46) -> (-5.08, 27.46) centre (-6.35, 27.46) ccw
  arc A630 (-7.62, 27.46) -> (-5.08, 27.46) centre (-6.35, 27.46) ccw
  arc A631 (-5.08, 27.46) -> (-7.62, 27.46) centre (-6.35, 27.46) ccw
  arc A632 (-5.08, 27.46) -> (-7.62, 27.46) centre (-6.35, 27.46) ccw
  arc A633 (-7.62, 27.46) -> (-5.08, 27.46) centre (-6.35, 27.46) ccw
  arc A634 (28.73, 30) -> (31.27, 30) centre (30, 30) ccw
  arc A635 (31.27, 30) -> (28.73, 30) centre (30, 30) ccw
  arc A636 (28.73, 30) -> (31.27, 30) centre (30, 30) ccw
  arc A637 (31.27, 30) -> (28.73, 30) centre (30, 30) ccw
  arc A638 (31.27, 30) -> (28.73, 30) centre (30, 30) ccw
  arc A639 (28.73, 30) -> (31.27, 30) centre (30, 30) ccw
  arc A640 (24.92, 27.46) -> (22.38, 27.46) centre (23.65, 27.46) ccw
  arc A641 (22.38, 27.46) -> (24.92, 27.46) centre (23.65, 27.46) ccw
  arc A642 (22.38, 27.46) -> (24.92, 27.46) centre (23.65, 27.46) ccw
  arc A643 (24.92, 27.46) -> (22.38, 27.46) centre (23.65, 27.46) ccw
  arc A644 (24.92, 27.46) -> (22.38, 27.46) centre (23.65, 27.46) ccw
  arc A645 (22.38, 27.46) -> (24.92, 27.46) centre (23.65, 27.46) ccw
  arc A646 (-181.27, 0) -> (-178.73, 0) centre (-180, 0) ccw
  arc A647 (-178.73, 0) -> (-181.27, 0) centre (-180, 0) ccw
  arc A648 (-181.27, 0) -> (-178.73, 0) centre (-180, 0) ccw
  arc A649 (-178.73, 0) -> (-181.27, 0) centre (-180, 0) ccw
  arc A650 (-178.73, 0) -> (-181.27, 0) centre (-180, 0) ccw
  arc A651 (-181.27, 0) -> (-178.73, 0) centre (-180, 0) ccw
  arc A652 (-185.08, -2.54) -> (-187.62, -2.54) centre (-186.35, -2.54) ccw
  arc A653 (-187.62, -2.54) -> (-185.08, -2.54) centre (-186.35, -2.54) ccw
  arc A654 (-187.62, -2.54) -> (-185.08, -2.54) centre (-186.35, -2.54) ccw
  arc A655 (-185.08, -2.54) -> (-187.62, -2.54) centre (-186.35, -2.54) ccw
  arc A656 (-185.08, -2.54) -> (-187.62, -2.54) centre (-186.35, -2.54) ccw
  arc A657 (-187.62, -2.54) -> (-185.08, -2.54) centre (-186.35, -2.54) ccw
  arc A658 (-148.73, 0) -> (-151.27, 0) centre (-150, 0) ccw
  arc A659 (-151.27, 0) -> (-148.73, 0) centre (-150, 0) ccw
  arc A660 (-148.73, 0) -> (-151.27, 0) centre (-150, 0) ccw
  arc A661 (-151.27, 0) -> (-148.73, 0) centre (-150, 0) ccw
  arc A662 (-148.73, 0) -> (-151.27, 0) centre (-150, 0) ccw
  arc A663 (-151.27, 0) -> (-148.73, 0) centre (-150, 0) ccw
  arc A664 (-157.62, -2.54) -> (-155.08, -2.54) centre (-156.35, -2.54) ccw
  arc A665 (-155.08, -2.54) -> (-157.62, -2.54) centre (-156.35, -2.54) ccw
  arc A666 (-157.62, -2.54) -> (-155.08, -2.54) centre (-156.35, -2.54) ccw
  arc A667 (-155.08, -2.54) -> (-157.62, -2.54) centre (-156.35, -2.54) ccw
  arc A668 (-155.08, -2.54) -> (-157.62, -2.54) centre (-156.35, -2.54) ccw
  arc A669 (-157.62, -2.54) -> (-155.08, -2.54) centre (-156.35, -2.54) ccw
  arc A670 (-121.27, 0) -> (-118.73, 0) centre (-120, 0) ccw
  arc A671 (-118.73, 0) -> (-121.27, 0) centre (-120, 0) ccw
  arc A672 (-118.73, 0) -> (-121.27, 0) centre (-120, 0) ccw
  arc A673 (-121.27, 0) -> (-118.73, 0) centre (-120, 0) ccw
  arc A674 (-118.73, 0) -> (-121.27, 0) centre (-120, 0) ccw
  arc A675 (-121.27, 0) -> (-118.73, 0) centre (-120, 0) ccw
  arc A676 (-127.62, -2.54) -> (-125.08, -2.54) centre (-126.35, -2.54) ccw
  arc A677 (-125.08, -2.54) -> (-127.62, -2.54) centre (-126.35, -2.54) ccw
  arc A678 (-127.62, -2.54) -> (-125.08, -2.54) centre (-126.35, -2.54) ccw
  arc A679 (-125.08, -2.54) -> (-127.62, -2.54) centre (-126.35, -2.54) ccw
  arc A680 (-127.62, -2.54) -> (-125.08, -2.54) centre (-126.35, -2.54) ccw
  arc A681 (-125.08, -2.54) -> (-127.62, -2.54) centre (-126.35, -2.54) ccw
  arc A682 (-88.73, 0) -> (-91.27, 0) centre (-90, 0) ccw
  arc A683 (-91.27, 0) -> (-88.73, 0) centre (-90, 0) ccw
  arc A684 (-91.27, 0) -> (-88.73, 0) centre (-90, 0) ccw
  arc A685 (-88.73, 0) -> (-91.27, 0) centre (-90, 0) ccw
  arc A686 (-91.27, 0) -> (-88.73, 0) centre (-90, 0) ccw
  arc A687 (-88.73, 0) -> (-91.27, 0) centre (-90, 0) ccw
  arc A688 (-97.62, -2.54) -> (-95.08, -2.54) centre (-96.35, -2.54) ccw
  arc A689 (-95.08, -2.54) -> (-97.62, -2.54) centre (-96.35, -2.54) ccw
  arc A690 (-97.62, -2.54) -> (-95.08, -2.54) centre (-96.35, -2.54) ccw
  arc A691 (-95.08, -2.54) -> (-97.62, -2.54) centre (-96.35, -2.54) ccw
  arc A692 (-95.08, -2.54) -> (-97.62, -2.54) centre (-96.35, -2.54) ccw
  arc A693 (-97.62, -2.54) -> (-95.08, -2.54) centre (-96.35, -2.54) ccw
  arc A694 (-58.73, 0) -> (-61.27, 0) centre (-60, 0) ccw
  arc A695 (-61.27, 0) -> (-58.73, 0) centre (-60, 0) ccw
  arc A696 (-61.27, 0) -> (-58.73, 0) centre (-60, 0) ccw
  arc A697 (-58.73, 0) -> (-61.27, 0) centre (-60, 0) ccw
  arc A698 (-61.27, 0) -> (-58.73, 0) centre (-60, 0) ccw
  arc A699 (-58.73, 0) -> (-61.27, 0) centre (-60, 0) ccw
  arc A700 (-65.08, -2.54) -> (-67.62, -2.54) centre (-66.35, -2.54) ccw
  arc A701 (-67.62, -2.54) -> (-65.08, -2.54) centre (-66.35, -2.54) ccw
  arc A702 (-65.08, -2.54) -> (-67.62, -2.54) centre (-66.35, -2.54) ccw
  arc A703 (-67.62, -2.54) -> (-65.08, -2.54) centre (-66.35, -2.54) ccw
  arc A704 (-67.62, -2.54) -> (-65.08, -2.54) centre (-66.35, -2.54) ccw
  arc A705 (-65.08, -2.54) -> (-67.62, -2.54) centre (-66.35, -2.54) ccw
  arc A706 (-31.27, 0) -> (-28.73, 0) centre (-30, 0) ccw
  arc A707 (-28.73, 0) -> (-31.27, 0) centre (-30, 0) ccw
  arc A708 (-28.73, 0) -> (-31.27, 0) centre (-30, 0) ccw
  arc A709 (-31.27, 0) -> (-28.73, 0) centre (-30, 0) ccw
  arc A710 (-31.27, 0) -> (-28.73, 0) centre (-30, 0) ccw
  arc A711 (-28.73, 0) -> (-31.27, 0) centre (-30, 0) ccw
  arc A712 (-35.08, -2.54) -> (-37.62, -2.54) centre (-36.35, -2.54) ccw
  arc A713 (-37.62, -2.54) -> (-35.08, -2.54) centre (-36.35, -2.54) ccw
  arc A714 (-37.62, -2.54) -> (-35.08, -2.54) centre (-36.35, -2.54) ccw
  arc A715 (-35.08, -2.54) -> (-37.62, -2.54) centre (-36.35, -2.54) ccw
  arc A716 (-35.08, -2.54) -> (-37.62, -2.54) centre (-36.35, -2.54) ccw
  arc A717 (-37.62, -2.54) -> (-35.08, -2.54) centre (-36.35, -2.54) ccw
  arc A718 (13.081, -0.254) -> (15.621, -0.254) centre (14.351, -0.254) ccw
  arc A719 (15.621, -0.254) -> (13.081, -0.254) centre (14.351, -0.254) ccw
  arc A720 (13.081, -0.254) -> (15.621, -0.254) centre (14.351, -0.254) ccw
  arc A721 (15.621, -0.254) -> (13.081, -0.254) centre (14.351, -0.254) ccw
  arc A722 (13.081, -0.254) -> (15.621, -0.254) centre (14.351, -0.254) ccw
  arc A723 (15.621, -0.254) -> (13.081, -0.254) centre (14.351, -0.254) ccw
  arc A724 (9.271, -2.794) -> (6.731, -2.794) centre (8.001, -2.794) ccw
  arc A725 (6.731, -2.794) -> (9.271, -2.794) centre (8.001, -2.794) ccw
  arc A726 (6.731, -2.794) -> (9.271, -2.794) centre (8.001, -2.794) ccw
  arc A727 (9.271, -2.794) -> (6.731, -2.794) centre (8.001, -2.794) ccw
  arc A728 (9.271, -2.794) -> (6.731, -2.794) centre (8.001, -2.794) ccw
  arc A729 (6.731, -2.794) -> (9.271, -2.794) centre (8.001, -2.794) ccw
  arc A730 (52.1971, -0.508) -> (54.7371, -0.508) centre (53.4671, -0.508) ccw
  arc A731 (54.7371, -0.508) -> (52.1971, -0.508) centre (53.4671, -0.508) ccw
  arc A732 (54.7371, -0.508) -> (52.1971, -0.508) centre (53.4671, -0.508) ccw
  arc A733 (52.1971, -0.508) -> (54.7371, -0.508) centre (53.4671, -0.508) ccw
  arc A734 (54.7371, -0.508) -> (52.1971, -0.508) centre (53.4671, -0.508) ccw
  arc A735 (52.1971, -0.508) -> (54.7371, -0.508) centre (53.4671, -0.508) ccw
  arc A736 (48.3871, -3.048) -> (45.8471, -3.048) centre (47.1171, -3.048) ccw
  arc A737 (45.8471, -3.048) -> (48.3871, -3.048) centre (47.1171, -3.048) ccw
  arc A738 (48.3871, -3.048) -> (45.8471, -3.048) centre (47.1171, -3.048) ccw
  arc A739 (45.8471, -3.048) -> (48.3871, -3.048) centre (47.1171, -3.048) ccw
  arc A740 (45.8471, -3.048) -> (48.3871, -3.048) centre (47.1171, -3.048) ccw
  arc A741 (48.3871, -3.048) -> (45.8471, -3.048) centre (47.1171, -3.048) ccw
  arc A742 (-193.49, -28.5751) -> (-190.95, -28.5751) centre (-192.22, -28.5751) ccw
  arc A743 (-190.95, -28.5751) -> (-193.49, -28.5751) centre (-192.22, -28.5751) ccw
  arc A744 (-193.49, -28.5751) -> (-190.95, -28.5751) centre (-192.22, -28.5751) ccw
  arc A745 (-190.95, -28.5751) -> (-193.49, -28.5751) centre (-192.22, -28.5751) ccw
  arc A746 (-193.49, -28.5751) -> (-190.95, -28.5751) centre (-192.22, -28.5751) ccw
  arc A747 (-190.95, -28.5751) -> (-193.49, -28.5751) centre (-192.22, -28.5751) ccw
  arc A748 (-197.3, -31.1151) -> (-199.84, -31.1151) centre (-198.57, -31.1151) ccw
  arc A749 (-199.84, -31.1151) -> (-197.3, -31.1151) centre (-198.57, -31.1151) ccw
  arc A750 (-199.84, -31.1151) -> (-197.3, -31.1151) centre (-198.57, -31.1151) ccw
  arc A751 (-197.3, -31.1151) -> (-199.84, -31.1151) centre (-198.57, -31.1151) ccw
  arc A752 (-197.3, -31.1151) -> (-199.84, -31.1151) centre (-198.57, -31.1151) ccw
  arc A753 (-199.84, -31.1151) -> (-197.3, -31.1151) centre (-198.57, -31.1151) ccw
  arc A754 (-163.49, -28.5751) -> (-160.95, -28.5751) centre (-162.22, -28.5751) ccw
  arc A755 (-160.95, -28.5751) -> (-163.49, -28.5751) centre (-162.22, -28.5751) ccw
  arc A756 (-163.49, -28.5751) -> (-160.95, -28.5751) centre (-162.22, -28.5751) ccw
  arc A757 (-160.95, -28.5751) -> (-163.49, -28.5751) centre (-162.22, -28.5751) ccw
  arc A758 (-163.49, -28.5751) -> (-160.95, -28.5751) centre (-162.22, -28.5751) ccw
  arc A759 (-160.95, -28.5751) -> (-163.49, -28.5751) centre (-162.22, -28.5751) ccw
  arc A760 (-169.84, -31.1151) -> (-167.3, -31.1151) centre (-168.57, -31.1151) ccw
  arc A761 (-167.3, -31.1151) -> (-169.84, -31.1151) centre (-168.57, -31.1151) ccw
  arc A762 (-167.3, -31.1151) -> (-169.84, -31.1151) centre (-168.57, -31.1151) ccw
  arc A763 (-169.84, -31.1151) -> (-167.3, -31.1151) centre (-168.57, -31.1151) ccw
  arc A764 (-167.3, -31.1151) -> (-169.84, -31.1151) centre (-168.57, -31.1151) ccw
  arc A765 (-169.84, -31.1151) -> (-167.3, -31.1151) centre (-168.57, -31.1151) ccw
  arc A766 (-133.49, -28.5751) -> (-130.95, -28.5751) centre (-132.22, -28.5751) ccw
  arc A767 (-130.95, -28.5751) -> (-133.49, -28.5751) centre (-132.22, -28.5751) ccw
  arc A768 (-133.49, -28.5751) -> (-130.95, -28.5751) centre (-132.22, -28.5751) ccw
  arc A769 (-130.95, -28.5751) -> (-133.49, -28.5751) centre (-132.22, -28.5751) ccw
  arc A770 (-133.49, -28.5751) -> (-130.95, -28.5751) centre (-132.22, -28.5751) ccw
  arc A771 (-130.95, -28.5751) -> (-133.49, -28.5751) centre (-132.22, -28.5751) ccw
  arc A772 (-139.84, -31.1151) -> (-137.3, -31.1151) centre (-138.57, -31.1151) ccw
  arc A773 (-137.3, -31.1151) -> (-139.84, -31.1151) centre (-138.57, -31.1151) ccw
  arc A774 (-137.3, -31.1151) -> (-139.84, -31.1151) centre (-138.57, -31.1151) ccw
  arc A775 (-139.84, -31.1151) -> (-137.3, -31.1151) centre (-138.57, -31.1151) ccw
  arc A776 (-139.84, -31.1151) -> (-137.3, -31.1151) centre (-138.57, -31.1151) ccw
  arc A777 (-137.3, -31.1151) -> (-139.84, -31.1151) centre (-138.57, -31.1151) ccw
  arc A778 (-100.95, -28.5751) -> (-103.49, -28.5751) centre (-102.22, -28.5751) ccw
  arc A779 (-103.49, -28.5751) -> (-100.95, -28.5751) centre (-102.22, -28.5751) ccw
  arc A780 (-100.95, -28.5751) -> (-103.49, -28.5751) centre (-102.22, -28.5751) ccw
  arc A781 (-103.49, -28.5751) -> (-100.95, -28.5751) centre (-102.22, -28.5751) ccw
  arc A782 (-100.95, -28.5751) -> (-103.49, -28.5751) centre (-102.22, -28.5751) ccw
  arc A783 (-103.49, -28.5751) -> (-100.95, -28.5751) centre (-102.22, -28.5751) ccw
  arc A784 (-109.84, -31.1151) -> (-107.3, -31.1151) centre (-108.57, -31.1151) ccw
  arc A785 (-107.3, -31.1151) -> (-109.84, -31.1151) centre (-108.57, -31.1151) ccw
  arc A786 (-107.3, -31.1151) -> (-109.84, -31.1151) centre (-108.57, -31.1151) ccw
  arc A787 (-109.84, -31.1151) -> (-107.3, -31.1151) centre (-108.57, -31.1151) ccw
  arc A788 (-109.84, -31.1151) -> (-107.3, -31.1151) centre (-108.57, -31.1151) ccw
  arc A789 (-107.3, -31.1151) -> (-109.84, -31.1151) centre (-108.57, -31.1151) ccw
  arc A790 (-70.95, -28.5751) -> (-73.49, -28.5751) centre (-72.22, -28.5751) ccw
  arc A791 (-73.49, -28.5751) -> (-70.95, -28.5751) centre (-72.22, -28.5751) ccw
  arc A792 (-70.95, -28.5751) -> (-73.49, -28.5751) centre (-72.22, -28.5751) ccw
  arc A793 (-73.49, -28.5751) -> (-70.95, -28.5751) centre (-72.22, -28.5751) ccw
  arc A794 (-70.95, -28.5751) -> (-73.49, -28.5751) centre (-72.22, -28.5751) ccw
  arc A795 (-73.49, -28.5751) -> (-70.95, -28.5751) centre (-72.22, -28.5751) ccw
  arc A796 (-79.84, -31.1151) -> (-77.3, -31.1151) centre (-78.57, -31.1151) ccw
  arc A797 (-77.3, -31.1151) -> (-79.84, -31.1151) centre (-78.57, -31.1151) ccw
  arc A798 (-79.84, -31.1151) -> (-77.3, -31.1151) centre (-78.57, -31.1151) ccw
  arc A799 (-77.3, -31.1151) -> (-79.84, -31.1151) centre (-78.57, -31.1151) ccw
  arc A800 (-79.84, -31.1151) -> (-77.3, -31.1151) centre (-78.57, -31.1151) ccw
  arc A801 (-77.3, -31.1151) -> (-79.84, -31.1151) centre (-78.57, -31.1151) ccw
  arc A802 (-43.49, -28.5751) -> (-40.95, -28.5751) centre (-42.22, -28.5751) ccw
  arc A803 (-40.95, -28.5751) -> (-43.49, -28.5751) centre (-42.22, -28.5751) ccw
  arc A804 (-43.49, -28.5751) -> (-40.95, -28.5751) centre (-42.22, -28.5751) ccw
  arc A805 (-40.95, -28.5751) -> (-43.49, -28.5751) centre (-42.22, -28.5751) ccw
  arc A806 (-40.95, -28.5751) -> (-43.49, -28.5751) centre (-42.22, -28.5751) ccw
  arc A807 (-43.49, -28.5751) -> (-40.95, -28.5751) centre (-42.22, -28.5751) ccw
  arc A808 (-49.84, -31.1151) -> (-47.3, -31.1151) centre (-48.57, -31.1151) ccw
  arc A809 (-47.3, -31.1151) -> (-49.84, -31.1151) centre (-48.57, -31.1151) ccw
  arc A810 (-49.84, -31.1151) -> (-47.3, -31.1151) centre (-48.57, -31.1151) ccw
  arc A811 (-47.3, -31.1151) -> (-49.84, -31.1151) centre (-48.57, -31.1151) ccw
  arc A812 (-49.84, -31.1151) -> (-47.3, -31.1151) centre (-48.57, -31.1151) ccw
  arc A813 (-47.3, -31.1151) -> (-49.84, -31.1151) centre (-48.57, -31.1151) ccw
  arc A814 (-10.95, -28.5751) -> (-13.49, -28.5751) centre (-12.22, -28.5751) ccw
  arc A815 (-13.49, -28.5751) -> (-10.95, -28.5751) centre (-12.22, -28.5751) ccw
  arc A816 (-10.95, -28.5751) -> (-13.49, -28.5751) centre (-12.22, -28.5751) ccw
  arc A817 (-13.49, -28.5751) -> (-10.95, -28.5751) centre (-12.22, -28.5751) ccw
  arc A818 (-10.95, -28.5751) -> (-13.49, -28.5751) centre (-12.22, -28.5751) ccw
  arc A819 (-13.49, -28.5751) -> (-10.95, -28.5751) centre (-12.22, -28.5751) ccw
  arc A820 (-19.84, -31.1151) -> (-17.3, -31.1151) centre (-18.57, -31.1151) ccw
  arc A821 (-17.3, -31.1151) -> (-19.84, -31.1151) centre (-18.57, -31.1151) ccw
  arc A822 (-17.3, -31.1151) -> (-19.84, -31.1151) centre (-18.57, -31.1151) ccw
  arc A823 (-19.84, -31.1151) -> (-17.3, -31.1151) centre (-18.57, -31.1151) ccw
  arc A824 (-19.84, -31.1151) -> (-17.3, -31.1151) centre (-18.57, -31.1151) ccw
  arc A825 (-17.3, -31.1151) -> (-19.84, -31.1151) centre (-18.57, -31.1151) ccw
  arc A826 (16.51, -28.5751) -> (19.05, -28.5751) centre (17.78, -28.5751) ccw
  arc A827 (19.05, -28.5751) -> (16.51, -28.5751) centre (17.78, -28.5751) ccw
  arc A828 (16.51, -28.5751) -> (19.05, -28.5751) centre (17.78, -28.5751) ccw
  arc A829 (19.05, -28.5751) -> (16.51, -28.5751) centre (17.78, -28.5751) ccw
  arc A830 (19.05, -28.5751) -> (16.51, -28.5751) centre (17.78, -28.5751) ccw
  arc A831 (16.51, -28.5751) -> (19.05, -28.5751) centre (17.78, -28.5751) ccw
  arc A832 (12.7, -31.1151) -> (10.16, -31.1151) centre (11.43, -31.1151) ccw
  arc A833 (10.16, -31.1151) -> (12.7, -31.1151) centre (11.43, -31.1151) ccw
  arc A834 (10.16, -31.1151) -> (12.7, -31.1151) centre (11.43, -31.1151) ccw
  arc A835 (12.7, -31.1151) -> (10.16, -31.1151) centre (11.43, -31.1151) ccw
  arc A836 (10.16, -31.1151) -> (12.7, -31.1151) centre (11.43, -31.1151) ccw
  arc A837 (12.7, -31.1151) -> (10.16, -31.1151) centre (11.43, -31.1151) ccw
  arc A838 (52.1946, -29.5911) -> (54.7346, -29.5911) centre (53.4646, -29.5911) ccw
  arc A839 (54.7346, -29.5911) -> (52.1946, -29.5911) centre (53.4646, -29.5911) ccw
  arc A840 (54.7346, -29.5911) -> (52.1946, -29.5911) centre (53.4646, -29.5911) ccw
  arc A841 (52.1946, -29.5911) -> (54.7346, -29.5911) centre (53.4646, -29.5911) ccw
  arc A842 (52.1946, -29.5911) -> (54.7346, -29.5911) centre (53.4646, -29.5911) ccw
  arc A843 (54.7346, -29.5911) -> (52.1946, -29.5911) centre (53.4646, -29.5911) ccw
  arc A844 (45.8446, -32.1311) -> (48.3846, -32.1311) centre (47.1146, -32.1311) ccw
  arc A845 (48.3846, -32.1311) -> (45.8446, -32.1311) centre (47.1146, -32.1311) ccw
  arc A846 (48.3846, -32.1311) -> (45.8446, -32.1311) centre (47.1146, -32.1311) ccw
  arc A847 (45.8446, -32.1311) -> (48.3846, -32.1311) centre (47.1146, -32.1311) ccw
  arc A848 (45.8446, -32.1311) -> (48.3846, -32.1311) centre (47.1146, -32.1311) ccw
  arc A849 (48.3846, -32.1311) -> (45.8446, -32.1311) centre (47.1146, -32.1311) ccw
  arc A850 (-186.7031, -55.6321) -> (-184.1631, -55.6321) centre (-185.4331, -55.6321) ccw
  arc A851 (-184.1631, -55.6321) -> (-186.7031, -55.6321) centre (-185.4331, -55.6321) ccw
  arc A852 (-184.1631, -55.6321) -> (-186.7031, -55.6321) centre (-185.4331, -55.6321) ccw
  arc A853 (-186.7031, -55.6321) -> (-184.1631, -55.6321) centre (-185.4331, -55.6321) ccw
  arc A854 (-184.1631, -55.6321) -> (-186.7031, -55.6321) centre (-185.4331, -55.6321) ccw
  arc A855 (-186.7031, -55.6321) -> (-184.1631, -55.6321) centre (-185.4331, -55.6321) ccw
  arc A856 (-190.5131, -58.1721) -> (-193.0531, -58.1721) centre (-191.7831, -58.1721) ccw
  arc A857 (-193.0531, -58.1721) -> (-190.5131, -58.1721) centre (-191.7831, -58.1721) ccw
  arc A858 (-190.5131, -58.1721) -> (-193.0531, -58.1721) centre (-191.7831, -58.1721) ccw
  arc A859 (-193.0531, -58.1721) -> (-190.5131, -58.1721) centre (-191.7831, -58.1721) ccw
  arc A860 (-190.5131, -58.1721) -> (-193.0531, -58.1721) centre (-191.7831, -58.1721) ccw
  arc A861 (-193.0531, -58.1721) -> (-190.5131, -58.1721) centre (-191.7831, -58.1721) ccw
  arc A862 (-156.7031, -55.6321) -> (-154.1631, -55.6321) centre (-155.4331, -55.6321) ccw
  arc A863 (-154.1631, -55.6321) -> (-156.7031, -55.6321) centre (-155.4331, -55.6321) ccw
  arc A864 (-154.1631, -55.6321) -> (-156.7031, -55.6321) centre (-155.4331, -55.6321) ccw
  arc A865 (-156.7031, -55.6321) -> (-154.1631, -55.6321) centre (-155.4331, -55.6321) ccw
  arc A866 (-156.7031, -55.6321) -> (-154.1631, -55.6321) centre (-155.4331, -55.6321) ccw
  arc A867 (-154.1631, -55.6321) -> (-156.7031, -55.6321) centre (-155.4331, -55.6321) ccw
  arc A868 (-163.0531, -58.1721) -> (-160.5131, -58.1721) centre (-161.7831, -58.1721) ccw
  arc A869 (-160.5131, -58.1721) -> (-163.0531, -58.1721) centre (-161.7831, -58.1721) ccw
  arc A870 (-163.0531, -58.1721) -> (-160.5131, -58.1721) centre (-161.7831, -58.1721) ccw
  arc A871 (-160.5131, -58.1721) -> (-163.0531, -58.1721) centre (-161.7831, -58.1721) ccw
  arc A872 (-160.5131, -58.1721) -> (-163.0531, -58.1721) centre (-161.7831, -58.1721) ccw